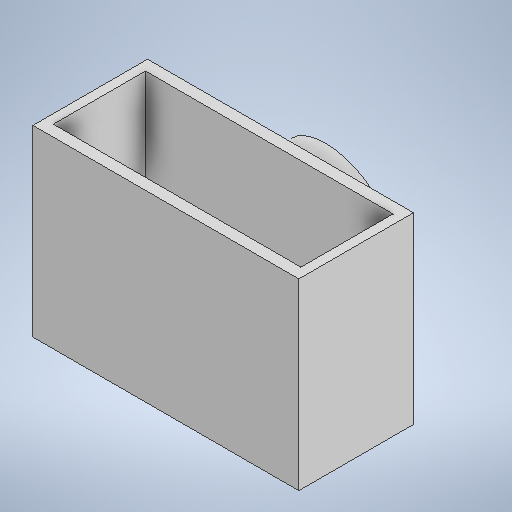
# Autodesk Inventor part: Attache servomoteur
Saved by Autodesk Inventor 2026.2 (Build 302298010, 298A)
## iProperties
Created: 2026-03-22
Part Number: Attache servomoteur
Material: Générique
Document SubType Name: Modeling
Designer: Genon
Density: 1 g/cm^3
Appearance: Par défaut
Author: Genon
Autodesk Inventor part; units mm, degrees
ref_plane "YZ Plane" through (0, 0, 0) normal (1, 0, 0) x (0, 1, 0)
ref_plane "XZ Plane" through (0, 0, 0) normal (0, 1, 0) x (-1, 0, 0)
ref_plane "XY Plane" through (0, 0, 0) normal (0, 0, 1) x (1, 0, 0)
sketch "Esquisse1" plane through (0, 0, 0) normal (0, 1, 0) x (-1, 0, 0)
  line L0 (0, 0) -> (29, 0)
  line L1 (29, 0) -> (29, 25)
  line L2 (29, 25) -> (-29, 25)
  line L3 (-29, 25) -> (-29, 0)
  line L4 (-29, 0) -> (0, 0)
  line L5 (0, 0) -> (0, 2.45)
  line L6 (0, 2.45) -> (27, 2.45)
  line L7 (27, 2.45) -> (27, 22.55)
  line L8 (27, 22.55) -> (-27, 22.55)
  line L9 (-27, 22.55) -> (-27, 2.45)
  line L10 (-27, 2.45) -> (0, 2.45)
  dimension "d0" = 29
  dimension "d1" = 25
  dimension "d2" = 58
  dimension "d3" = 29
  dimension "d4" = 2.45
  dimension "d5" = 27
  dimension "d7" = 20.1
  dimension "d8" = 54
  constraints: 22 end point, 7 perpendicular, 2 vertical, 1 horizontal, 1 parallel, 1 point on line
  measures "d0" distance of L0.start L0.end
  measures "d1" distance of L0.end L1.end
  measures "d2" distance of L1.end L2.end
  measures "d3" distance of L3.end L0.start
  measures "d4" distance of L0.start L5.end
  measures "d5" distance of L5.end L6.end
  measures "d7" distance of L6.end L7.end
  measures "d8" distance of L7.end L8.end
extrude "Extrusion1" add sketch "Esquisse1" along normal blind 40
ref_plane "Plan de construction1" through (0, 0, 0) normal (0, 0.2046669, -0.9788317) x (1, 0, 0)
sketch "Esquisse2" plane through (0, 0, 0) normal (0, 0.2046669, -0.9788317) x (1, 0, 0)
  line L0 (0, 0) -> (0, -20)
  circle A0 centre (0, -20) radius 10
  circle A1 centre (0, -20) radius 11
  dimension "d12" = 20
  dimension "d13" = 20
  dimension "d14" = 22
  constraints: 2 centre point, 2 coincident, 2 end point, 1 vertical
  measures "d12" distance of L0.start L0.end
  measures "d13" diameter of A0
  measures "d14" diameter of A1
extrude "Extrusion2" add sketch "Esquisse2" along normal blind 16.5
sketch "Esquisse3" plane through (0, 40, 0) normal (0, 1, 0) x (1, 0, 0)
  line L0 (-27, -22.55) -> (-27, -2.45) projected
  line L1 (27, -22.55) -> (-27, -22.55) projected
  line L2 (-27, -2.45) -> (27, -2.45) projected
  line L3 (27, -2.45) -> (27, -22.55) projected
  point P0 (0, 0)
extrude "Extrusion3" cut sketch "Esquisse3" against normal through all
ref_plane "Plan de construction2" through (0, 1.3303, -6.3624) normal (0, 0.2046669, -0.9788317) x (1, 0, 0)
sketch "Esquisse4" plane through (0, 1.3303, -6.3624) normal (0, 0.2046669, -0.9788317) x (1, 0, 0)
  circle A0 centre (0, -20) radius 10 projected
  point P0 (0, 0)
extrude "Extrusion4" add sketch "Esquisse4" against normal blind 2
ref_plane "Plan de construction3" through (29, 0, 0) normal (0, -0.9788317, -0.2046669) x (-1, 0, 0)
sketch "Esquisse5" plane through (29, 0, 0) normal (0, -0.9788317, -0.2046669) x (-1, 0, 0)
  line L0 (40, 16.5) -> (18, 16.5) projected
  line L1 (29, 16.5) -> (29, 11.5)
  point P0 (29, 0)
  dimension "d23" = 5
  constraints: 2 end point, 1 coincident, 1 midpoint, 1 vertical
  measures "d23" distance of L1.start L1.end
hole "Perçage1" at (0, 2.3537, -11.2566) direction (0, 0.9788317, 0.2046669) diameter 4 end through all
sketch "Esquisse6" plane through (0, 0, 0) normal (0, -1, 0) x (1, 0, 0)
  line L0 (27, 2.45) -> (27, 22.55) projected
  line L1 (-27, 22.55) -> (-27, 2.45) projected
  line L2 (27, 22.55) -> (21, 22.55)
  line L3 (27, 22.55) -> (-27, 22.55) projected
  line L4 (21, 22.55) -> (21, 2.45)
  line L5 (21, 2.45) -> (27, 2.45)
  line L6 (-27, 22.55) -> (-21, 22.55)
  line L7 (-21, 22.55) -> (-21, 2.45)
  line L8 (-21, 2.45) -> (-27, 2.45)
  point P0 (0, 0)
  dimension "d31" = 6
  dimension "d32" = 6
  constraints: 12 end point, 4 perpendicular, 3 point on line
  measures "d31" distance of L0.end L2.end
  measures "d32" distance of L1.start L6.end
extrude "Extrusion5" add sketch "Esquisse6" against normal blind 16.4
sketch "Esquisse7" plane through (0, 16.4, 0) normal (0, 1, 0) x (1, 0, 0)
  line L0 (-27, -22.55) -> (-27, -2.45) projected
  line L1 (-27, -12.5) -> (-24.775, -12.5)
  line L2 (-24.775, -12.5) -> (-24.775, -17.5)
  line L3 (-24.775, -12.5) -> (-24.775, -7.5)
  line L4 (27, -2.45) -> (27, -22.55) projected
  line L5 (27, -22.55) -> (27, -12.5)
  line L6 (27, -12.5) -> (24.775, -12.5)
  line L7 (24.775, -12.5) -> (24.775, -7.5)
  line L8 (21, -22.55) -> (21, -2.45) projected
  line L9 (24.775, -12.5) -> (24.775, -17.5)
  point P0 (0, 0)
  dimension "d35" = 2.225
  dimension "d36" = 5
  dimension "d37" = 5
  dimension "d38" = 2.225
  dimension "d39" = 5
  dimension "d41" = 5
  constraints: 14 end point, 4 coincident, 3 perpendicular, 2 midpoint, 2 vertical, 1 horizontal
  measures "d35" distance of L1.start L1.end
  measures "d36" distance of L1.end L2.end
  measures "d37" distance of L1.end L3.end
  measures "d38" distance of L5.end L6.end
  measures "d39" distance of L6.end L7.end
  measures "d41" distance of L6.end L9.end
hole "Perçage2" at (-24.775, 16.4, 17.5) at (-24.775, 16.4, 7.5) at (24.775, 16.4, 17.5) at (24.775, 16.4, 7.5) direction (0, -1, 0) diameter 3.242 depth 11.8 tip angle 118 thread size "M4x0.7" class "6H" standard "ISO Metric profile"
sketch "Esquisse8" plane through (0, 16.4, 0) normal (0, 1, 0) x (1, 0, 0)
  line L0 (-21, -22.55) -> (-21, -2.45) projected
  line L1 (-27, -22.55) -> (-27, -2.45) projected
  line L2 (-27, -12.5) -> (-27, -11.5)
  line L3 (-27, -11.5) -> (-21, -11.5)
  line L4 (-27, -12.5) -> (-27, -13.5)
  line L5 (-27, -13.5) -> (-21, -13.5)
  line L6 (-21, -11.5) -> (-21, -13.5)
  line L7 (21, -2.45) -> (21, -22.55) projected
  line L8 (27, -2.45) -> (27, -22.55) projected
  line L9 (27, -22.55) -> (27, -12.5)
  line L10 (27, -12.5) -> (27, -11.5)
  line L11 (21, -11.5) -> (27, -11.5)
  line L12 (21, -11.5) -> (21, -13.5)
  line L13 (21, -13.5) -> (27, -13.5)
  point P0 (0, 0)
  dimension "d49" = 1
  dimension "d50" = 1
  dimension "d54" = 10.05
  dimension "d55" = 6
  dimension "d56" = 2
  dimension "d57" = 1
  constraints: 20 end point, 8 point on line, 5 perpendicular, 3 midpoint
  measures "d49" distance of L2.start L2.end
  measures "d50" distance of L2.start L4.end
  measures "d54" distance of L8.end L9.end
  measures "d55" distance of L11.start L10.end
  measures "d56" distance of L11.start L12.end
  measures "d57" distance of L13.end point (27, -12.5)
extrude "Extrusion6" cut sketch "Esquisse8" against normal blind 2
